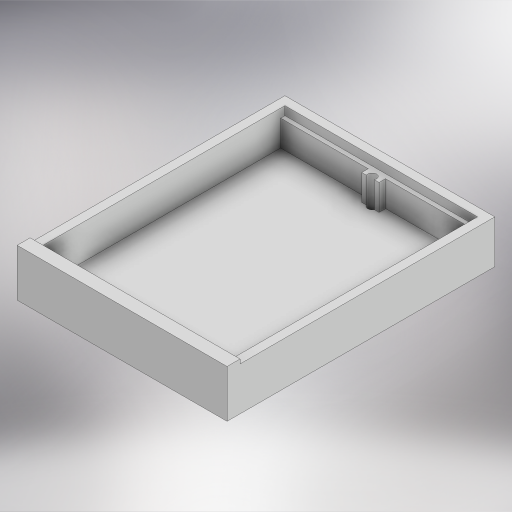
# Autodesk Inventor part: Module Cover
Saved by Autodesk Inventor 2024 (Build 280153000, 153)
## iProperties
Created: 2023-10-04
Part Number: Module Cover
Material: Generic
Document SubType Name: Modeling
Designer: cfang
Density: 1 g/cm^3
Appearance: Default
Author: cfang
Autodesk Inventor part; units mm, degrees
ref_plane "YZ Plane" through (0, 0, 0) normal (1, 0, 0) x (0, 1, 0)
ref_plane "XZ Plane" through (0, 0, 0) normal (0, 1, 0) x (-1, 0, 0)
ref_plane "XY Plane" through (0, 0, 0) normal (0, 0, 1) x (1, 0, 0)
sketch "Sketch1" plane through (0, 0, 0) normal (0, 1, 0) x (-1, 0, 0)
  line L0 (-24.3, -31) -> (24.3, -31)
  line L1 (24.3, -31) -> (24.3, 31)
  line L2 (24.3, 31) -> (-24.3, 31)
  line L3 (-24.3, 31) -> (-24.3, -31)
  line L4 (-24.3, -31) -> (24.3, 31) construction
  line L5 (24.3, -31) -> (-24.3, 31) construction
  point P0 (0, 0)
  dimension "d0" = 62
  dimension "d1" = 48.6
  constraints: 12 end point, 2 midpoint, 2 parallel, 1 horizontal, 1 perpendicular
  measures "d0" distance of L0.end L1.end
  measures "d1" distance of L1.end L2.end
extrude "Extrusion1" add sketch "Sketch1" along normal blind 10
sketch "Sketch2" plane through (0, 10, 0) normal (0, 1, 0) x (1, 0, 0)
  line L0 (22.3, 29) -> (-22.3, 29)
  line L1 (-22.3, 29) -> (-22.3, -29)
  line L2 (-22.3, -29) -> (22.3, -29)
  line L3 (22.3, -29) -> (22.3, 29)
  line L4 (22.3, 29) -> (-22.3, -29) construction
  line L5 (-22.3, 29) -> (22.3, -29) construction
  line L6 (-24.3, 31) -> (-24.3, -31) projected
  line L7 (-24.3, -31) -> (24.3, -31) projected
  point P0 (0, 0)
  dimension "d4" = 2
  dimension "d5" = 2
  constraints: 12 end point, 2 midpoint, 2 parallel, 1 horizontal, 1 perpendicular
  measures "d4" distance between parallel lines of L6 L1
  measures "d5" distance between parallel lines of L7 L2
extrude "Extrusion2" cut sketch "Sketch2" against normal blind 2
sketch "Sketch3" plane through (0, 8, 0) normal (0, 1, 0) x (1, 0, 0)
  line L0 (-22.3, -29) -> (-22.3, 29) projected
  line L1 (22.3, 28) -> (-22.3, 28)
  line L2 (-22.3, 28) -> (-22.3, -28)
  line L3 (-22.3, -28) -> (22.3, -28)
  line L4 (22.3, -28) -> (22.3, 28)
  line L5 (22.3, 28) -> (-22.3, -28) construction
  line L6 (-22.3, 28) -> (22.3, -28) construction
  line L7 (22.3, -29) -> (-22.3, -29) projected
  point P0 (0, 0)
  dimension "d8" = 1
  constraints: 12 end point, 2 midpoint, 2 parallel, 1 horizontal, 1 perpendicular, 1 point on line
  measures "d8" distance between parallel lines of L3 L7
extrude "Extrusion3" cut sketch "Sketch3" against normal blind 6
sketch "Sketch4" plane through (24.3, 0, 31) normal (1, 0, 0) x (0, 0, -1)
  line L0 (62, 10) -> (0, 10) projected
  line L1 (0, 10) -> (3, 10)
  line L2 (3, 10) -> (3, 11)
  line L3 (3, 11) -> (0, 11)
  line L4 (0, 11) -> (0, 10)
  point P0 (31, 0)
  point P1 (3, 10)
  dimension "d11" = 3
  dimension "d12" = 1
  constraints: 8 end point, 2 parallel, 1 horizontal, 1 perpendicular
  measures "d11" distance of L3.end L2.end
  measures "d12" distance of L2.end L1.end
extrude "Extrusion4" add sketch "Sketch4" against normal up to surface (48.6 mm away)
sketch "Sketch6" plane through (0, 8, 0) normal (0, 1, 0) x (1, 0, 0)
  line L0 (-22.3, 28) -> (22.3, 28) projected
  line L1 (2, 28) -> (-2, 28)
  line L2 (-2, 28) -> (-2, 26.5)
  line L3 (-2, 26.5) -> (2, 26.5)
  line L4 (2, 26.5) -> (2, 28)
  point P0 (0, 0)
  dimension "d15" = 4
  dimension "d16" = 2
  dimension "d17" = 1.5
  constraints: 8 end point, 2 parallel, 1 horizontal, 1 perpendicular, 1 point on line
  measures "d15" distance of L2.end L3.end
  measures "d16" distance from line of L2 point (0, 0)
  measures "d17" distance of L3.end L1.start
extrude "Extrusion5" add sketch "Sketch6" against normal up to surface (6 mm away)
sketch "Sketch7" plane through (0, 8, 0) normal (0, 1, 0) x (1, 0, 0)
  line L0 (-22.3, 29) -> (22.3, 29) projected
  point P0 (0, 0)
  point P1 (0, 26.9)
  dimension "d20" = 2.1
  measures "d20" distance from line of L0 point (0, 26.9)
hole "Hole1" at (0, 8, -26.9) direction (0, -1, 0) diameter 2 end through all
equation "\"d5\" = d4"
equation "\"d16\" = 0.5 * d15"
body "Solid1"
